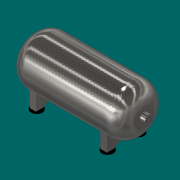
# Autodesk Inventor part: Part1
Saved by Autodesk Inventor 2017 (Build 210142000, 142)
## iProperties
Created: 2020-05-05
Part Number: Part1
Material: Generic
Document SubType Name: Sheet Metal
Designer: IVAN
Density: 1 g/cm^3
Sheet Metal Rule: Default
Appearance: Default
Author: IVAN
Autodesk Inventor part; units mm, degrees
ref_plane "YZ Plane" through (0, 0, 0) normal (1, 0, 0) x (0, 1, 0)
ref_plane "XZ Plane" through (0, 0, 0) normal (0, 1, 0) x (-1, 0, 0)
ref_plane "XY Plane" through (0, 0, 0) normal (0, 0, 1) x (1, 0, 0)
sketch "Sketch2" plane through (0, 0, 0) normal (1, 0, 0) x (0, 1, 0)
  circle A0 centre (0, 0) radius 75
  dimension "d2" = 150
  constraints: 1 centre point, 1 coincident
  measures "d2" diameter of A0
extrude "Extrusion1" add sketch "Sketch2" along normal mid plane 350
fillet "Fillet1" radius 50 2 edges at (-175, -75, 0) (175, -75, 0)
sketch "Sketch3" plane through (175, 0, 0) normal (1, 0, 0) x (0, 0, -1)
  circle A0 centre (0, 0) radius 12.5
  dimension "d6" = 25
  constraints: 1 centre point, 1 coincident
  measures "d6" diameter of A0
extrude "Extrusion2" add sketch "Sketch3" along normal blind 15
sketch "Sketch4" plane through (0, 0, 0) normal (0, 1, 0) x (-1, 0, 0)
  line L0 (120, 60) -> (100, 60)
  line L1 (100, 60) -> (100, -60)
  line L2 (100, -60) -> (120, -60)
  line L3 (120, -60) -> (120, 60)
  line L4 (120, 60) -> (100, -60) construction
  line L5 (100, 60) -> (120, -60) construction
  point P0 (0, 0)
  point P1 (110, 0)
  dimension "d9" = 20
  dimension "d10" = 120
  constraints: 12 end point, 2 midpoint, 2 parallel, 1 horizontal, 1 perpendicular
  measures "d9" distance of L2.end L1.end
  measures "d10" distance of L1.end L0.end
extrude "Extrusion3" add sketch "Sketch4" against normal blind 94
mirror "Mirror1" about plane through (0, 0, 0) normal (1, 0, 0) of "Extrusion3"
sketch "Sketch5" plane through (-120, -94, -60) normal (-1, 0, 0) x (0, 0, 1)
  line L0 (0, 0) -> (120, 0) projected
  line L1 (0, 0) -> (25, 0)
  line L2 (25, 0) -> (25, 15)
  line L3 (25, 15) -> (0, 15)
  line L4 (0, 15) -> (0, 0)
  line L5 (95, 15) -> (120, 15)
  line L6 (120, 15) -> (120, 0)
  line L7 (120, 0) -> (95, 0)
  line L8 (95, 0) -> (95, 15)
  arc A0 (95, 0) -> (25, 0) centre (60, -33.3333) ccw
  line L9 (25, 0) -> (95, 0)
  point P0 (60, 94)
  dimension "d13" = 25
  dimension "d14" = 15
  dimension "d15" = 25
  constraints: 18 end point, 4 parallel, 2 horizontal, 2 perpendicular, 2 point on circle, 1 centre point, 1 collinear, 1 point on line
  measures "d13" distance of L3.end L2.end
  measures "d14" distance of L2.end L1.end
  measures "d15" distance of L5.start L5.end
extrude "Extrusion4" cut sketch "Sketch5" against normal up to surface (240 mm away) contours A0 L0
sketch "Sketch7" plane through (0, -94, 0) normal (0, -1, 0) x (1, 0, 0)
  line L0 (-120, 35) -> (-100, 35) projected
  line L1 (-100, 35) -> (-100, 60) projected
  line L2 (-100, 60) -> (-120, 60) projected
  line L3 (-120, 60) -> (-120, 35) projected
  circle A0 centre (-110, 47.5) radius 17.5
  point P0 (0, 0)
  dimension "d18" = 35
  constraints: 1 centre point
  measures "d18" diameter of A0
extrude "Extrusion5" add sketch "Sketch7" along normal blind 5 contours L3 L2 L1 L0 | A0
mirror "Mirror2" about plane through (0, 0, 0) normal (0, 0, 1) of "Extrusion5"
mirror "Mirror3" about plane through (0, 0, 0) normal (1, 0, 0) of "Extrusion5", "Mirror2"
equation "\"d15\" = d13"
equation "\"BendRadius\" = Thickness"
equation "\"BendReliefWidth\" = Thickness"
equation "\"BendReliefDepth\" = 0.5 * Thickness"
equation "\"CornerReliefSize\" = 4 * Thickness"
equation "\"MinimumRemnant\" = 2 * Thickness"
equation "\"TransitionRadius\" = BendRadius"
equation "\"JacobiRadiusSize\" = BendRadius"
equation "\"GapSize\" = Thickness"
equation "\"Thickness\" = 3.048"
body "Solid1"
